Autodesk Fusion 360 part; units mm, degrees
(part 2 of 5)
sketch "Sketch1 (8)" plane through (0, 0, 0) normal (0, 0, 1) x (1, 0, 0) in component "main-switchbody (2)"
  line L0 (0, 0) -> (0, 20) construction
  line L1 (0, 20) -> (20, 20) construction
  line L2 (20, 20) -> (20, 0) construction
  line L3 (20, 0) -> (0, 0) construction
  line L4 (0, 0) -> (20, 20) construction
  line L5 (20, 0) -> (0, 20) construction
  line L6 (10, 0) -> (18.9, 0) construction
  line L7 (10, 10) -> (18.9, 10) construction
  line L8 (18.9, 10) -> (18.9, 18.9) construction
  line L9 (18.9, 18.9) -> (1.1, 18.9) construction
  line L10 (1.1, 18.9) -> (1.1, 1.1) construction
  line L11 (1.1, 1.1) -> (18.9, 1.1) construction
  line L12 (18.9, 1.1) -> (18.9, 18.9) construction
  line L13 (10, 10) -> (3.05, 10) construction
  line L14 (3.05, 10) -> (3.05, 16.95) construction
  line L15 (3.05, 16.95) -> (16.95, 16.95) construction
  line L16 (16.95, 16.95) -> (16.95, 3.05) construction
  line L17 (16.95, 3.05) -> (3.05, 3.05) construction
  line L18 (3.05, 3.05) -> (3.05, 16.95) construction
  line L19 (3.05, 3.05) -> (0, 3.05) construction
  line L20 (3.05, 3.05) -> (3.05, 0) construction
  line L21 (16.95, 3.05) -> (20, 3.05) construction
  line L22 (16.95, 16.95) -> (20, 16.95) construction
  line L23 (16.95, 16.95) -> (16.95, 20) construction
  line L24 (3.05, 16.95) -> (3.05, 20) construction
  line L25 (3.05, 16.95) -> (0, 16.95) construction
  line L26 (3.05, 18.9) -> (6.05, 18.9) construction
  line L27 (6.05, 18.9) -> (6.05, 20) construction
  line L28 (16.95, 18.9) -> (13.95, 18.9) construction
  line L29 (13.95, 18.9) -> (13.95, 20) construction
  line L30 (16.95, 3.05) -> (16.95, 0) construction
  line L31 (16.95, 1.1) -> (13.95, 1.1) construction
  line L32 (13.95, 1.1) -> (13.95, 0) construction
  line L33 (3.05, 1.1) -> (6.05, 1.1) construction
  line L34 (6.05, 1.1) -> (6.05, 0) construction
  line L35 (0, 20) -> (20, 20) construction
  line L36 (20, 20) -> (20, 0) construction
  line L37 (20, 0) -> (0, 0) construction
  line L38 (0, 0) -> (0, 20) construction
  line L39 (0, 20) -> (20, 20)
  line L40 (20, 20) -> (20, 0)
  line L41 (20, 0) -> (0, 0)
  line L42 (0, 0) -> (0, 20)
  line L43 (16.95, 3.05) -> (3.05, 3.05)
  line L44 (3.05, 3.05) -> (3.05, 16.95)
  line L45 (3.05, 16.95) -> (16.95, 16.95)
  line L46 (16.95, 16.95) -> (16.95, 3.05)
  line L47 (3.05, 1.1) -> (6.05, 1.1)
  line L48 (6.05, 1.1) -> (6.05, 0)
  line L49 (6.05, 0) -> (3.05, 0)
  line L50 (3.05, 0) -> (3.05, 1.1)
  line L51 (13.95, 1.1) -> (16.95, 1.1)
  line L52 (16.95, 1.1) -> (16.95, 0)
  line L53 (16.95, 0) -> (13.95, 0)
  line L54 (13.95, 0) -> (13.95, 1.1)
  line L55 (13.95, 20) -> (16.95, 20)
  line L56 (16.95, 20) -> (16.95, 18.9)
  line L57 (16.95, 18.9) -> (13.95, 18.9)
  line L58 (13.95, 18.9) -> (13.95, 20)
  line L59 (3.05, 20) -> (6.05, 20)
  line L60 (6.05, 20) -> (6.05, 18.9)
  line L61 (6.05, 18.9) -> (3.05, 18.9)
  line L62 (3.05, 18.9) -> (3.05, 20)
  line L63 (1.1, 10) -> (1.1, 12)
  line L64 (1.1, 10) -> (1.1, 8)
  line L65 (1.1, 8) -> (-1.9, 8)
  line L66 (-1.9, 8) -> (1.1, 8)
  line L67 (1.1, 8) -> (1.1, 12)
  line L68 (1.1, 12) -> (-1.9, 12)
  line L69 (-1.9, 12) -> (-1.9, 8)
  line L70 (3.05, 10) -> (3.05, 7.5) construction
  line L71 (3.05, 7.5) -> (2.55, 7.5) construction
  line L72 (2.55, 7.5) -> (2.55, 12.5) construction
  line L73 (2.55, 12.5) -> (3.05, 12.5085) construction
  line L74 (3.05, 12.5085) -> (3.05, 7.5) construction
  line L75 (2.55, 12.5) -> (16.95, 12.5) construction
  line L76 (16.95, 12.5) -> (17.45, 12.5) construction
  line L77 (17.45, 12.5) -> (17.45, 7.5) construction
  line L78 (17.45, 7.5) -> (16.95, 7.5) construction
  line L79 (16.95, 7.5) -> (16.95, 12.5) construction
  line L80 (17.45, 7.5) -> (16.95, 7.5)
  line L81 (16.95, 7.5) -> (16.95, 12.5)
  line L82 (16.95, 12.5) -> (17.45, 12.5)
  line L83 (17.45, 12.5) -> (17.45, 7.5)
  line L84 (3.05, 7.5) -> (2.55, 7.5)
  line L85 (2.55, 7.5) -> (2.55, 12.5)
  line L86 (2.55, 12.5) -> (3.05, 12.5)
  line L87 (3.05, 12.5) -> (3.05, 7.5)
  dimension "d1_2" = 20
  dimension "d2_2" = 20
  dimension "d3_2" = 8.9
  dimension "d4_2" = 8.9
  dimension "d5_2" = 8.9
  dimension "d6_2" = 17.8
  dimension "d7_2" = 17.8
  dimension "d8_2" = 6.95
  dimension "d9_2" = 6.95
  dimension "d10_2" = 13.9
  dimension "d11_2" = 13.9
  dimension "d12_2" = 13.9
  dimension "d13_2" = 3
  dimension "d14_2" = 3
  dimension "d15_2" = 3
  dimension "d16_2" = 3
  dimension "d21_4" = 3
  dimension "d58_4" = 2.5
  dimension "d59_4" = 0.5
  dimension "d60_4" = 5
  dimension "d61_4" = 0.5
  dimension "d62_4" = 5
  constraint coincident L0.start L3.end
  constraint vertical L0
  constraint perpendicular L0 L1
  constraint perpendicular L1 L2
  constraint perpendicular L0 L3
  constraint midpoint L3 L6.start
  constraint parallel L3 L6
  constraint midpoint L4 L7.start
  constraint parallel L6 L7
  constraint perpendicular L7 L8
  constraint perpendicular L8 L9
  constraint perpendicular L9 L10
  constraint coincident L5 L11.end
  constraint perpendicular L10 L11
  constraint perpendicular L12 L13
  constraint perpendicular L13 L14
  constraint perpendicular L14 L15
  constraint perpendicular L7 L16
  constraint perpendicular L16 L17
  constraint coincident L0 L19.end
  constraint perpendicular L0 L19
  constraint coincident L3 L20.end
  constraint perpendicular L3 L20
  constraint coincident L2 L21.end
  constraint perpendicular L2 L21
  constraint coincident L2 L22.end
  constraint perpendicular L2 L22
  constraint coincident L1 L23.end
  constraint perpendicular L1 L23
  constraint coincident L1 L24.end
  constraint perpendicular L1 L24
  constraint coincident L0 L25.end
  constraint perpendicular L0 L25
  constraint coincident L24 L26.start
  constraint coincident L9 L26.start
  constraint coincident L9 L26.end
  constraint coincident L1 L27.end
  constraint perpendicular L1 L27
  constraint coincident L9 L28.start
  constraint coincident L23 L28.start
  constraint perpendicular L23 L28
  constraint coincident L1 L29.end
  constraint perpendicular L1 L29
  constraint coincident L6 L30.end
  constraint coincident L30 L31.start
  constraint coincident L11 L31.start
  constraint perpendicular L30 L31
  constraint coincident L6 L32.end
  constraint coincident L11 L33.start
  constraint coincident L20 L33.start
  constraint perpendicular L20 L33
  constraint coincident L3 L34.end
  constraint perpendicular L3 L34
  constraint horizontal L35
  constraint vertical L36
  constraint horizontal L37
  constraint vertical L38
  constraint horizontal L39
  constraint vertical L40
  constraint horizontal L41
  constraint vertical L42
  constraint horizontal L43
  constraint vertical L44
  constraint horizontal L45
  constraint vertical L46
  constraint horizontal L47
  constraint vertical L48
  constraint horizontal L49
  constraint vertical L50
  constraint horizontal L51
  constraint vertical L52
  constraint horizontal L53
  constraint vertical L54
  constraint horizontal L55
  constraint vertical L56
  constraint horizontal L57
  constraint vertical L58
  constraint horizontal L59
  constraint vertical L60
  constraint horizontal L61
  constraint vertical L62
  constraint midpoint L10 L63.start
  constraint coincident L10 L63.end
  constraint parallel L10 L63
  constraint coincident L10 L64.end
  constraint perpendicular L0 L65
  constraint horizontal L66
  constraint vertical L67
  constraint horizontal L68
  constraint vertical L69
  constraint perpendicular L13 L70
  constraint perpendicular L70 L71
  constraint perpendicular L71 L72
  constraint coincident L14 L73.end
  constraint perpendicular L71 L74
  constraint coincident L16 L75.end
  constraint perpendicular L16 L75
  constraint perpendicular L16 L76
  constraint perpendicular L76 L77
  constraint coincident L16 L78.end
  constraint perpendicular L16 L78
  constraint horizontal L80
  constraint vertical L81
  constraint horizontal L82
  constraint vertical L83
  constraint horizontal L84
  constraint vertical L85
  constraint horizontal L86
  constraint vertical L87
  measures "d1_2" distance of L0.start L0.end
  measures "d2_2" distance of L0.end L1.end
  measures "d3_2" distance of L6.start L6.end
  measures "d4_2" distance of L7.start L7.end
  measures "d5_2" distance of L7.end L8.end
  measures "d6_2" distance of L8.end L9.end
  measures "d7_2" distance of L9.end L10.end
  measures "d8_2" distance of L7.start L13.end
  measures "d9_2" distance of L13.end L14.end
  measures "d10_2" distance of L14.end L15.end
  measures "d11_2" distance of L15.end L16.end
  measures "d12_2" distance of L16.end L17.end
  measures "d13_2" distance of L26.start L26.end
  measures "d14_2" distance of L28.start L28.end
  measures "d15_2" distance of L31.start L31.end
  measures "d16_2" distance of L33.start L33.end
  measures "d21_4" distance of L64.end L65.end
  measures "d58_4" distance of L13.end L70.end
  measures "d59_4" distance of L70.end L71.end
  measures "d60_4" distance of L71.end L72.end
  measures "d61_4" distance of L75.end L76.end
  measures "d62_4" distance of L76.end L77.end
extrude "Extrude3'''" add sketch "Sketch1 (8)" along normal blind 7.5 separate body contours L42 L63 L64 L65 L66 L67 L68 | L42 L65 L66 L68 L69 makes body 11 in component "main-switchbody (2)"
extrude "Extrude2'''" add sketch "Sketch1 (8)" along normal blind 4 separate body contours L39 L40 L41 L42 L47 L48 L50 L51 L52 L54 L56 L57 L58 L60 L61 L62 L63 L64 L65 L66 L67 L68 | L42 L63 L64 L65 L66 L67 L68 | L46 L80 L81 L82 L83 | L44 L84 L85 L86 L87 makes body 12 in component "main-switchbody (2)"
extrude "Extrude1'''''" add sketch "Sketch1 (8)" along normal blind 6 separate body contours L39 L59 L60 L61 L62 | L39 L55 L56 L57 L58 | L41 L47 L48 L49 L50 | L41 L51 L52 L53 L54 makes body 13 at (4.05, 1.1, 2) makes body 14 at (5.05, 20, 4) makes body 15 at (14.95, 1.1, 2) makes body 16 at (14.95, 20, 2) in component "main-switchbody (2)"
extrude "Extrude4'" cut sketch "Sketch1 (8)" along normal blind 2 contours L42 L65 L66 L68 L69 bodies 11 in component "main-switchbody (2)"
sketch "Sketch2 (6)" plane through (1.1, 0, 0) normal (1, 0, 0) x (0, 1, 0) in component "main-switchbody (2)"
  line L0 (8, 0) -> (12, 0)
  line L1 (12, 0) -> (12, 7.5)
  line L2 (12, 7.5) -> (8, 7.5)
  line L3 (8, 7.5) -> (8, 0)
  line L4 (8, 7.5) -> (8, 4) construction
  line L5 (8, 4) -> (12, 4) construction
  line L6 (12, 4) -> (12, 7.5) construction
  line L7 (12, 7.5) -> (8, 7.5) construction
  line L8 (8, 7.5) -> (8, 5.75) construction
  line L9 (8, 5.75) -> (12, 5.75) construction
  line L10 (8, 7.5) -> (12, 7.5)
  line L11 (12, 7.5) -> (12, 5.75)
  line L12 (12, 5.75) -> (8, 5.75)
  line L13 (8, 5.75) -> (8, 7.5)
  dimension "d26_4" = 1.75
  constraint coincident L2.end L3.start
  constraint coincident L3 L4.end
  constraint perpendicular L2 L4
  constraint coincident L1 L5.end
  constraint perpendicular L1 L5
  constraint coincident L1.end L2.start
  constraint perpendicular L2 L6
  constraint perpendicular L5 L8
  constraint midpoint L6 L9.end
  constraint horizontal L10
  constraint vertical L11
  constraint horizontal L12
  constraint vertical L13
  measures "d26_4" distance of L2.end L8.end
extrude "Extrude5'" add sketch "Sketch2 (6)" along normal blind 1 contours L1 L2 L3 L10 L11 L12 L13 bodies 11 in component "main-switchbody (2)"
extrude "Extrude6'" cut 1 faces at (-1.9, 10.6667, 3.8333) along direction (1, 0, 0) blind 1 on bodies 11 bodies 11 in component "main-switchbody (2)"
sketch "Sketch3 (2)" plane through (0, 18.9, 0) normal (0, -1, 0) x (1, 0, 0) in component "main-switchbody (2)"
  line L0 (3.05, 0) -> (6.05, 0)
  line L1 (6.05, 0) -> (6.05, 6)
  line L2 (6.05, 6) -> (3.05, 6)
  line L3 (3.05, 6) -> (3.05, 0)
  line L4 (3.05, 6) -> (3.05, 4) construction
  line L5 (6.05, 4) -> (6.05, 6) construction
  line L6 (3.05, 6) -> (3.05, 4.5) construction
  line L7 (6.05, 6) -> (6.05, 4.5) construction
  arc A0 (6.05, 4.5) -> (3.05, 4.5) centre (4.55, 4.5) ccw construction
  arc A1 (6.05, 4.5) -> (3.05, 4.5) centre (4.55, 4.5) ccw
  dimension "d31_4" = 1.5
  dimension "d32_4" = 1.5
  constraint coincident L2.end L3.start
  constraint coincident L3 L4.end
  constraint perpendicular L2 L4
  constraint coincident L1 L5.start
  constraint coincident L1.end L2.start
  constraint perpendicular L2 L5
  constraint perpendicular L2 L6
  constraint perpendicular L2 L7
  constraint tangent L2 A0
  constraint tangent L2 A1
  measures "d31_4" distance of L2.end L6.end
  measures "d32_4" distance of L1.end L7.end
extrude "Extrude7'" cut sketch "Sketch3 (2)" against normal blind 1.1 contours L2 L3 A1 | L1 L2 A1 bodies 14 in component "main-switchbody (2)"
sketch "Sketch4 (2)" plane through (0, 0, 0) normal (0, -1, 0) x (1, 0, 0) in component "main-switchbody (2)"
  line L0 (3.05, 0) -> (6.05, 0)
  line L1 (6.05, 0) -> (6.05, 6)
  line L2 (6.05, 6) -> (3.05, 6)
  line L3 (3.05, 6) -> (3.05, 0)
  line L4 (3.05, 6) -> (3.05, 4.5) construction
  line L5 (6.05, 6) -> (6.05, 4.5) construction
  arc A0 (6.05, 4.5) -> (3.05, 4.5) centre (4.55, 4.5) ccw
  constraint coincident L2.end L3.start
  constraint coincident L3 L4.end
  constraint perpendicular L2 L4
  constraint coincident L1.end L2.start
  constraint coincident L1 L5.end
  constraint perpendicular L2 L5
  constraint tangent L2 A0
extrude "Extrude8'" cut sketch "Sketch4 (2)" against normal blind 1.1 contours L2 L3 A0 | L1 L2 A0 bodies 13 in component "main-switchbody (2)"
sketch "Sketch5 (2)" plane through (0, 0, 0) normal (0, -1, 0) x (1, 0, 0) in component "main-switchbody (2)"
  line L0 (13.95, 0) -> (16.95, 0)
  line L1 (16.95, 0) -> (16.95, 6)
  line L2 (16.95, 6) -> (13.95, 6)
  line L3 (13.95, 6) -> (13.95, 0)
  line L4 (13.95, 6) -> (13.95, 4.5) construction
  line L5 (16.95, 6) -> (16.95, 4.5) construction
  arc A0 (16.95, 4.5) -> (13.95, 4.5) centre (15.45, 4.5) ccw
  constraint coincident L2.end L3.start
  constraint coincident L3 L4.end
  constraint perpendicular L2 L4
  constraint coincident L1.end L2.start
  constraint coincident L1 L5.end
  constraint perpendicular L2 L5
  constraint tangent L2 A0
extrude "Extrude9'" cut sketch "Sketch5 (2)" against normal blind 1.1 contours L2 L3 A0 | L1 L2 A0 bodies 15 in component "main-switchbody (2)"
sketch "Sketch6 (2)" plane through (0, 18.9, 0) normal (0, -1, 0) x (1, 0, 0) in component "main-switchbody (2)"
  line L0 (13.95, 0) -> (16.95, 0)
  line L1 (16.95, 0) -> (16.95, 6)
  line L2 (16.95, 6) -> (13.95, 6)
  line L3 (13.95, 6) -> (13.95, 0)
  line L4 (13.95, 6) -> (13.95, 4.5) construction
  line L5 (16.95, 6) -> (16.95, 4.5) construction
  arc A0 (16.95, 4.5) -> (13.95, 4.5) centre (15.45, 4.5) ccw
  constraint coincident L2.end L3.start
  constraint coincident L3 L4.end
  constraint perpendicular L2 L4
  constraint coincident L1.end L2.start
  constraint coincident L1 L5.end
  constraint perpendicular L2 L5
  constraint tangent L2 A0
extrude "Extrude10'" cut sketch "Sketch6 (2)" against normal blind 1.1 contours L2 L3 A0 | L1 L2 A0 bodies 16 in component "main-switchbody (2)"
sketch "Sketch7 (2)" plane through (0, 0, 4) normal (0, 0, 1) x (-1, 0, 0) in component "main-switchbody (2)"
  line L0 (-3.05, -16.95) -> (-16.95, -16.95)
  line L1 (-16.95, -16.95) -> (-16.95, -3.05)
  line L2 (-16.95, -3.05) -> (-3.05, -3.05)
  line L3 (-3.05, -3.05) -> (-3.05, -16.95)
  line L4 (-6.05, -20) -> (-6.05, -18.9)
  line L5 (-6.05, -18.9) -> (-3.05, -18.9)
  line L6 (-3.05, -18.9) -> (-3.05, -20)
  line L7 (-3.05, -20) -> (0, -20)
  line L8 (0, -20) -> (0, 0)
  line L9 (0, 0) -> (-3.05, 0)
  line L10 (-3.05, 0) -> (-3.05, -1.1)
  line L11 (-3.05, -1.1) -> (-6.05, -1.1)
  line L12 (-6.05, -1.1) -> (-6.05, 0)
  line L13 (-6.05, 0) -> (-13.95, 0)
  line L14 (-13.95, 0) -> (-13.95, -1.1)
  line L15 (-13.95, -1.1) -> (-16.95, -1.1)
  line L16 (-16.95, -1.1) -> (-16.95, 0)
  line L17 (-16.95, 0) -> (-20, 0)
  line L18 (-20, 0) -> (-20, -20)
  line L19 (-20, -20) -> (-16.95, -20)
  line L20 (-16.95, -20) -> (-16.95, -18.9)
  line L21 (-16.95, -18.9) -> (-13.95, -18.9)
  line L22 (-13.95, -18.9) -> (-13.95, -20)
  line L23 (-13.95, -20) -> (-6.05, -20)
  line L24 (-20, -10) -> (-20, -11.5) construction
  line L25 (-20, -10) -> (-20, -8.5) construction
  line L26 (-20, -8.5) -> (-19, -8.5) construction
  line L27 (-19, -8.5) -> (-19, -11.5) construction
  line L28 (-19, -11.5) -> (-20, -11.5) construction
  line L29 (-20, -11.5) -> (-21, -11.5) construction
  line L30 (-21, -11.5) -> (-21, -8.5) construction
  line L31 (-21, -8.5) -> (-20, -8.5) construction
  line L32 (-19, -11.5) -> (-21, -11.5)
  line L33 (-21, -11.5) -> (-21, -8.5)
  line L34 (-21, -8.5) -> (-19, -8.5)
  line L35 (-19, -8.5) -> (-19, -11.5)
  dimension "d41_4" = 1.5
  dimension "d42_4" = 1
  constraint midpoint L18 L24.start
  constraint parallel L18 L24
  constraint coincident L18 L25.end
  constraint parallel L18 L25
  constraint perpendicular L25 L26
  constraint perpendicular L26 L27
  constraint perpendicular L24 L29
  constraint perpendicular L29 L30
  constraint horizontal L32
  constraint vertical L33
  constraint horizontal L34
  constraint vertical L35
  measures "d41_4" distance of L24.start L24.end
  measures "d42_4" distance of L24.end L29.end
extrude "Extrude11'" add sketch "Sketch7 (2)" along normal blind 3 contours L18 L32 L33 L34 | L18 L32 L34 L35 bodies 12 in component "main-switchbody (2)"
extrude "Extrude12'" add 1 faces at (20, 8.5, 6) along direction (0, -1, 0) blind 0.5 on bodies 12 bodies 12 in component "main-switchbody (2)"
extrude "Extrude13'" add 1 faces at (20, 11.5, 6) along direction (0, 1, 0) blind 0.5 on bodies 12 bodies 12 in component "main-switchbody (2)"
extrude "Extrude14'" add 1 faces at (20.3333, 10.6667, 7) along direction (0, 0, 1) blind 0.75 on bodies 12 bodies 12 in component "main-switchbody (2)"
sketch "Sketch8 (2)" plane through (0, 0, 4) normal (0, 0, -1) x (1, 0, 0) in component "main-switchbody (2)"
  line L0 (20, -8) -> (20, -12)
  line L1 (20, -12) -> (21, -12)
  line L2 (21, -12) -> (21, -8)
  line L3 (21, -8) -> (20, -8)
  line L4 (20, -12) -> (20, -8)
  constraint coincident L0.end L1.start
  constraint coincident L0.start L3.end
extrude "Extrude15'" add sketch "Sketch8 (2)" along normal blind 2 bodies 12 in component "main-switchbody (2)"
sketch "Sketch9 (3)" plane through (19, 0, 0) normal (-1, 0, 0) x (0, -1, 0) in component "main-switchbody (2)"
  line L0 (-12, 4) -> (-8, 4)
  line L1 (-8, 4) -> (-8, 7.75)
  line L2 (-8, 7.75) -> (-12, 7.75)
  line L3 (-12, 7.75) -> (-12, 4)
  line L4 (-12, 7.75) -> (-12, 5.75) construction
  line L5 (-12, 5.75) -> (-8, 5.75) construction
  line L6 (-12, 7.75) -> (-8, 7.75)
  line L7 (-8, 7.75) -> (-8, 5.75)
  line L8 (-8, 5.75) -> (-12, 5.75)
  line L9 (-12, 5.75) -> (-12, 7.75)
  dimension "d53_4" = 2
  constraint coincident L2.end L3.start
  constraint perpendicular L2 L4
  constraint coincident L1 L5.end
  constraint perpendicular L1 L5
  constraint horizontal L6
  constraint vertical L7
  constraint horizontal L8
  constraint vertical L9
  measures "d53_4" distance of L2.end L4.end
extrude "Extrude16'" add sketch "Sketch9 (3)" along normal blind 0.5 contours L1 L2 L3 L6 L7 L8 L9 bodies 12 in component "main-switchbody (2)"
extrude "Extrude17'" cut 1 faces at (2.1, 9.3333, 6.9167) along direction (-1, 0, 0) blind 0.3 on bodies 11 bodies 11 in component "main-switchbody (2)"
extrude "Extrude18'" cut sketch "Sketch1 (8)" along normal blind 2.7 contours L44 L84 L85 L86 L87 bodies 12 in component "main-switchbody (2)"
extrude "Extrude19'" cut sketch "Sketch1 (8)" along normal blind 2.7 contours L46 L80 L81 L82 L83 bodies 12 in component "main-switchbody (2)"
extrude "Extrude20'" add sketch "Sketch1 (8)" against normal blind 0.2 contours L39 L40 L41 L42 L47 L48 L50 L51 L52 L54 L56 L57 L58 L60 L61 L62 L63 L64 L65 L66 L67 L68 | L39 L59 L60 L61 L62 | L42 L63 L64 L65 L66 L67 L68 | L39 L55 L56 L57 L58 | L41 L47 L48 L49 L50 | L41 L51 L52 L53 L54 bodies 11 12 13 14 15 16 in component "main-switchbody (2)"
fillet "Fillet1'" radius 1 2 edges at (21, 10, 7.75) (-0.9, 10, 7.5) on bodies 11 12 in component "main-switchbody (2)"
extrude "Extrude21'" add 1 faces at (2.8833, 9.1667, 2.7) along direction (0, 0, -1) blind 2.9 on bodies 11 bodies 11 in component "main-switchbody (2)"
extrude "Extrude22'" add 1 faces at (17.1167, 10.8333, 2.7) along direction (0, 0, -1) blind 2.9 on bodies 11 bodies 11 in component "main-switchbody (2)"
sketch "Sketch10 (2)" plane through (0, 0, 4) normal (0, 0, 1) x (-1, 0, 0) in component "main-switchbody (2)"
  line L0 (-3.05, -16.95) -> (-16.95, -16.95)
  line L1 (-16.95, -16.95) -> (-16.95, -3.05)
  line L2 (-16.95, -3.05) -> (-3.05, -3.05)
  line L3 (-3.05, -3.05) -> (-3.05, -16.95)
  line L4 (0, -12) -> (-1.1, -12)
  line L5 (-1.1, -12) -> (-1.1, -8)
  line L6 (-1.1, -8) -> (0, -8)
  line L7 (0, -8) -> (0, 0)
  line L8 (0, 0) -> (-3.05, 0)
  line L9 (-3.05, 0) -> (-3.05, -1.1)
  line L10 (-3.05, -1.1) -> (-6.05, -1.1)
  line L11 (-6.05, -1.1) -> (-6.05, 0)
  line L12 (-6.05, 0) -> (-13.95, 0)
  line L13 (-13.95, 0) -> (-13.95, -1.1)
  line L14 (-13.95, -1.1) -> (-16.95, -1.1)
  line L15 (-16.95, -1.1) -> (-16.95, 0)
  line L16 (-16.95, 0) -> (-20, 0)
  line L17 (-20, 0) -> (-20, -8)
  line L18 (-20, -8) -> (-19, -8)
  line L19 (-19, -8) -> (-19, -12)
  line L20 (-19, -12) -> (-20, -12)
  line L21 (-20, -12) -> (-20, -20)
  line L22 (-20, -20) -> (-16.95, -20)
  line L23 (-16.95, -20) -> (-16.95, -18.9)
  line L24 (-16.95, -18.9) -> (-13.95, -18.9)
  line L25 (-13.95, -18.9) -> (-13.95, -20)
  line L26 (-13.95, -20) -> (-6.05, -20)
  line L27 (-6.05, -20) -> (-6.05, -18.9)
  line L28 (-6.05, -18.9) -> (-3.05, -18.9)
  line L29 (-3.05, -18.9) -> (-3.05, -20)
  line L30 (-3.05, -20) -> (0, -20)
  line L31 (0, -20) -> (0, -12)
  line L32 (-3.05, -10) -> (-3.05, -12.5) construction
  line L33 (-3.05, -12.5) -> (-3.05, -7.5) construction
  line L34 (-3.05, -7.5) -> (-2.55, -7.5) construction
  line L35 (-2.55, -7.5) -> (-3.05, -7.5) construction
  line L36 (-3.05, -7.5) -> (-3.05, -12.5) construction
  line L37 (-3.05, -12.5) -> (-2.55, -12.5) construction
  line L38 (-2.55, -12.5) -> (-2.55, -7.5) construction
  line L39 (-3.05, -12.5) -> (-16.95, -12.5) construction
  line L40 (-16.95, -12.5) -> (-16.95, -7.5) construction
  line L41 (-16.95, -7.5) -> (-17.45, -7.5) construction
  line L42 (-17.45, -7.5) -> (-16.95, -7.5) construction
  line L43 (-16.95, -7.5) -> (-16.95, -12.5) construction
  line L44 (-16.95, -12.5) -> (-17.45, -12.5) construction
  line L45 (-17.45, -12.5) -> (-17.45, -7.5) construction
  line L46 (-16.95, -12.5) -> (-17.45, -12.5)
  line L47 (-17.45, -12.5) -> (-17.45, -7.5)
  line L48 (-17.45, -7.5) -> (-16.95, -7.5)
  line L49 (-16.95, -7.5) -> (-16.95, -12.5)
  line L50 (-2.55, -12.5) -> (-3.05, -12.5)
  line L51 (-3.05, -12.5) -> (-3.05, -7.5)
  line L52 (-3.05, -7.5) -> (-2.55, -7.5)
  line L53 (-2.55, -7.5) -> (-2.55, -12.5)
  dimension "d75_2" = 5
  dimension "d76_2" = 0.5
  dimension "d77_2" = 0.5
  constraint midpoint L3 L32.start
  constraint coincident L3 L32.end
  constraint perpendicular L0 L32
  constraint parallel L3 L33
  constraint perpendicular L33 L34
  constraint horizontal L35
  constraint vertical L36
  constraint horizontal L37
  constraint vertical L38
  constraint coincident L1 L39.end
  constraint perpendicular L1 L39
  constraint coincident L1 L40.end
  constraint perpendicular L39 L40
  constraint perpendicular L40 L41
  constraint horizontal L42
  constraint vertical L43
  constraint horizontal L44
  constraint vertical L45
  constraint horizontal L46
  constraint vertical L47
  constraint horizontal L48
  constraint vertical L49
  constraint horizontal L50
  constraint vertical L51
  constraint horizontal L52
  constraint vertical L53
  measures "d75_2" distance of L32.end L33.end
  measures "d76_2" distance of L33.end L34.end
  measures "d77_2" distance of L40.end L41.end
extrude "Extrude23'" cut sketch "Sketch10 (2)" against normal blind 2.9 contours L3 L50 L51 L52 L53 | L1 L46 L47 L48 L49 bodies 11 in component "main-switchbody (2)"
extrude "Extrude24'" cut 2 faces at (4.8122, 18.9, 5.1079) (15.1626, 18.9, 5.4316) along direction (0, 1, 0) blind 0.25 on bodies 11 bodies 11 in component "main-switchbody (2)"
extrude "Extrude25'" cut 2 faces at (4.2822, 1.1, 5.1824) (15.2673, 1.1, 4.9654) along direction (0, -1, 0) blind 0.25 on bodies 11 bodies 11 in component "main-switchbody (2)"
extrude "Extrude26'" add 1 faces at (1.0167, 12.3167, -0.2) along direction (0, 0, -1) blind 1 on bodies 11 bodies 11 in component "main-switchbody (2)"
extrude "Extrude27'" cut 1 faces at (1.0167, 12.3167, -1.2) along direction (0, 0, 1) blind 0.2 on bodies 11 bodies 11 in component "main-switchbody (2)"
extrude "Extrude28'" cut 2 faces at (17.1167, 10.8333, 1.1) (2.8833, 9.1667, 1.1) along direction (0, 0, -1) blind 0.8 on bodies 11 bodies 11 in component "main-switchbody (2)"
extrude "Extrude29'" cut 1 faces at (18.8333, 9.3333, 5.75) along direction (0, 0, 1) blind 0.2 on bodies 11 bodies 11 in component "main-switchbody (2)"
extrude "Extrude30'" cut 1 faces at (1.3333, 10.6667, 5.75) along direction (0, 0, 1) blind 0.2 on bodies 11 bodies 11 in component "main-switchbody (2)"
sketch "Sketch1 (9)" plane through (0, 0, 0.0152) normal (0, 0, -1) x (1, 0, 0) in component "mxledbit-switchbody v10 (2)"
  line L0 (4.5419, -16.2374) -> (4.5419, -2.3374)
  line L1 (4.5419, -2.3374) -> (18.4419, -2.3374)
  line L2 (18.4419, -2.3374) -> (18.4419, -16.2374)
  line L3 (18.4419, -16.2374) -> (4.5419, -16.2374)
  line L4 (1.4919, -19.2874) -> (21.4919, -19.2874)
  line L5 (21.4919, -19.2874) -> (21.4919, 0.7126)
  line L6 (21.4919, 0.7126) -> (1.4919, 0.7126)
  line L7 (1.4919, 0.7126) -> (1.4919, -19.2874)
ref_plane "WorkPlane1" through (5, 31.8794, 9.316) normal (0, -0.939693, 0.34202) x (1, 0, 0) in component "wheel (1)"
sketch "Sketch2 (7)" plane through (5, 31.8794, 9.316) normal (0, -0.939693, 0.34202) x (1, 0, 0) in component "wheel (1)"
  circle A0 centre (0, 0) radius 80
  dimension "d64_1" = 160
  constraint coincident A0.centre origin
  measures "d64_1" diameter of A0
component_pattern "component pattern'" in component "Index2"
sketch "Sketch2 (8)" plane through (0, 23.2767, -8.472) normal (0, -0.939693, 0.34202) x (1, 0, 0) in component "IND-Sketch (1)"
  circle A0 centre (5, 19.6575) radius 80
  line L0 (5, 19.6575) -> (5, -60.3425) construction
  line L1 (5, -60.3425) -> (-10, -60.3425) construction
  line L2 (-10, -60.3425) -> (20, -60.3425)
  line L3 (20, -60.3425) -> (20, 19.6575)
  line L4 (20, 19.6575) -> (-10, 19.6575)
  line L5 (-10, 19.6575) -> (-10, -60.3425)
  dimension "d69_1" = 80
  dimension "d70_1" = 15
  dimension "d71_1" = 30
  dimension "d72_1" = 80
  constraint coincident A0.centre L0.start
  constraint vertical L0
  constraint perpendicular L0 L1
  constraint horizontal L2
  constraint vertical L3
  constraint horizontal L4
  constraint vertical L5
  measures "d69_1" distance of A0.centre L0.end
  measures "d70_1" distance of L0.end L1.end
  measures "d71_1" distance of L1.end L2.end
  measures "d72_1" distance of L1.end L4.end
sketch "Sketch9 (4)" plane through (5, 41.9534, 55.6343) normal (0, 0.573576, 0.819152) x (-1, 0, 0) in component "IND-Sketch (1)"
  line L0 (-45, -9.823) -> (5, -9.823) construction
  line L1 (-20, -9.823) -> (5, -9.823) construction
  line L2 (-20, -9.823) -> (-45, -9.823) construction
  circle A0 centre (-20, -9.823) radius 75 construction
  point P0 (-20, -9.823)
  point P1 (-45, -9.823)
  point P2 (5, -9.823)
  point P3 (5, -9.823)
  point P4 (-45, -9.823)
  dimension "d38_1" = 30
  dimension "d39_1" = 15
  dimension "d40_1" = 15
  dimension "d41_1" = 160
  constraint coincident P4 P1
  constraint horizontal L0
  constraint coincident P0 L1.start
  constraint parallel L0 L1
  constraint parallel L0 L2
sketch "Sketch1 (10)" plane through (0, 54.7581, -45.9475) normal (0, -0.766044, 0.642788) x (1, 0, 0) in component "IND-Sketch (1)"
  line L0 (-1.3269, 70.632) -> (-1.3269, 84.532)
  line L1 (-1.3269, 84.532) -> (12.5731, 84.532)
  line L2 (12.5731, 84.532) -> (12.5731, 70.632)
  line L3 (12.5731, 70.632) -> (-1.3269, 70.632)
  line L4 (-4.3769, 67.582) -> (15.6231, 67.582)
  line L5 (15.6231, 67.582) -> (15.6231, 87.582)
  line L6 (15.6231, 87.582) -> (-4.3769, 87.582)
  line L7 (-4.3769, 87.582) -> (-4.3769, 67.582)
  line L8 (-4.3769, 77.582) -> (15.6231, 77.582) construction
  line L9 (5.6231, 87.582) -> (5.6231, 67.582) construction
  point P0 (5.6231, 77.582)
  constraint midpoint L7 L8.start
  constraint midpoint L5 L8.end
  constraint midpoint L6 L9.start
  constraint midpoint L4 L9.end
  constraint midpoint L8 P0
ref_plane "WorkPlane2" through (0, 34, 0) normal (0, 1, 0) x (0, 0, 1) in component "IND-Sketch (2)"
sketch "IND-originXY (3)" plane through (0, 0, 0) normal (0, 0, 1) x (1, 0, 0) in component "IND-Sketch (2)"
  line L0 (0, 0) -> (0, 16) construction
  line L1 (0, 16) -> (16, 16) construction
  line L2 (16, 16) -> (16, -18) construction
  line L3 (16, -18) -> (-18, -18) construction
  line L4 (0, 16) -> (17, 16) construction
  point P0 (17, 16)
  dimension "d20_3" = 16
  dimension "d21_3" = 16
  dimension "d29_3" = 34
  dimension "d30_3" = 34
  dimension "d34_3" = 17
  constraint coincident L0.start origin
  constraint vertical L0
  constraint perpendicular L0 L1
  constraint perpendicular L1 L2
  constraint perpendicular L0 L3
  constraint perpendicular L0 L4
  constraint coincident P0 L4.end
  measures "d20_3" distance of L0.start L0.end
  measures "d21_3" distance of L0.end L1.end
  measures "d29_3" distance of L1.end L2.end
  measures "d30_3" distance of L2.end L3.end
  measures "d34_3" distance of L0.end P0
sketch "IND-originXZ (3)" plane through (0, 34, 0) normal (0, 1, 0) x (1, 0, 0) in component "IND-Sketch (2)"
  line L0 (0, 0) -> (16, 0) construction
  line L1 (10, 0) -> (10, -10) construction
  line L2 (10, -10) -> (0, -10) construction
  line L3 (0, -10) -> (0, 0) construction
  line L4 (10, -10) -> (5, -10) construction
  line L5 (0, -10) -> (5, -10) construction
  line L6 (0, -10) -> (5, -10) construction
  point P0 (16, 0)
  point P1 (0, -10)
  point P2 (10, -10)
  point P3 (17, 0)
  point P4 (5, -10)
  dimension "d26_3" = 10
  dimension "d27_3" = 34
  dimension "d28_3" = 34
  dimension "d36_3" = 17
  dimension "d37_3" = 17
  constraint coincident P0 L1.start
  constraint perpendicular L0 L1
  constraint perpendicular L1 L2
  constraint coincident L0.start L3.end
  constraint coincident P1 L2.end
  constraint coincident P2 L1.end
  constraint midpoint L2 P4
  constraint perpendicular L1 L4
  constraint parallel L4 L6
  measures "d26_3" distance of L1.start P2
ref_plane "WorkPlane3" through (5, 34, 10) normal (0, 0.996195, -0.087156) x (-1, 0, 0) in component "IND-Sketch (2)"
sketch "IND-path (3)" plane through (5, 34.1975, 12.2574) normal (0, 0.996195, -0.087156) x (-1, 0, 0) in component "IND-Sketch (2)"
  line L0 (-5, -2.266) -> (5, -2.266) construction
  line L1 (5, -2.266) -> (-5, -2.266) construction
  circle A0 centre (0, 0) radius 85 construction
  line L2 (0, 0) -> (17, 0) construction
  line L3 (0, 0) -> (-17, 0) construction
  line L4 (0, 0) -> (0, -85) construction
  line L5 (0, -85) -> (6.95, -85) construction
  line L6 (0, -85) -> (-6.95, -85) construction
  point P0 (-5, -2.266)
  point P1 (5, -2.266)
  point P2 (0, -85)
  dimension "d32_3" = 170
  dimension "d33_3" = 17
  dimension "d35_3" = 17
  dimension "d42_3" = 85
  dimension "d43_3" = 6.95
  dimension "d44_3" = 6.95
  dimension "d67_3" = 90
  constraint coincident P1 L0.end
  constraint coincident P0 L0.start
  constraint coincident A0.centre L2.start
  constraint parallel L1 L2
  constraint parallel L0 L3
  constraint coincident P2 L4.end
  constraint perpendicular L4 L5
  constraint perpendicular L4 L6
  measures "d32_3" diameter of A0
  measures "d33_3" distance of A0.centre L2.end
  measures "d35_3" distance of A0.centre L3.end
  measures "d42_3" distance of A0.centre P2
  measures "d43_3" distance of P2 L5.end
  measures "d44_3" distance of P2 L6.end
  measures "d67_3" angle of L2 L4
sketch "Sketch1 (11)" plane through (5, 34.1975, 12.2574) normal (0, 0.996195, -0.087156) x (-1, 0, 0) in component "wheel (2)"
  circle A0 centre (0, 0) radius 85
  line L0 (0, -85) -> (6.95, -85)
  line L1 (0, -85) -> (-6.95, -85)
  line L2 (0, -85) -> (0, 85) construction
  line L3 (0, 0) -> (85, 0) construction
  circle A1 centre (0, 0) radius 85
  point P0 (0, -85)
  point P1 (0, -2.266)
  dimension "d45_3" = 170
  dimension "d46_3" = 85
  dimension "d47_3" = 170
  constraint coincident P0 L0.start
  constraint perpendicular L0 L2
  constraint coincident A0.centre L3.start
  constraint perpendicular L2 L3
  measures "d45_3" distance of P0 L2.end
  measures "d46_3" distance of A0.centre L3.end
  measures "d47_3" diameter of A1
extrude "Extrude1''''''" add sketch "Sketch1 (11)" along normal blind 4 separate body makes body 17 in component "wheel (2)"
ref_plane "WorkPlane1" through (5, 50.9494, -74.5329) normal (0, -0.087156, -0.996195) x (1, 0, 0) in component "plug (2)"
sketch "Sketch1 (12)" plane through (5, 73.9095, -76.5416) normal (0, -0.087156, -0.996195) x (1, 0, 0) in component "plug (2)"
  line L0 (-85, 43.3002) -> (85, 43.3002)
  line L1 (-85, 43.3002) -> (85, 43.3002)
  line L2 (-85, 47.3002) -> (85, 47.3002)
  line L3 (-85, 47.3002) -> (85, 47.3002)
  line L4 (0, 47.3002) -> (0, 43.3002) construction
  line L5 (0, 47.3002) -> (-6.95, 47.3002) construction
  line L6 (0, 47.3002) -> (6.95, 47.3002) construction
  line L7 (6.95, 47.3002) -> (6.95, 43.3002) construction
  line L8 (-6.95, 47.3002) -> (-6.95, 43.3002) construction
  line L9 (-6.95, 43.3002) -> (6.95, 43.3002) construction
  line L10 (6.95, 43.3002) -> (-6.95, 43.3002)
  line L11 (-6.95, 43.3002) -> (-6.95, 47.3002)
  line L12 (-6.95, 47.3002) -> (6.95, 47.3002)
  line L13 (6.95, 47.3002) -> (6.95, 43.3002)
  point P0 (0, 47.3002)
  dimension "d51_3" = 6.95
  dimension "d52_3" = 6.95
  constraint coincident P0 L4.start
  constraint midpoint L1 L4.end
  constraint perpendicular L4 L5
  constraint perpendicular L4 L6
  constraint coincident L1 L7.end
  constraint perpendicular L1 L7
  constraint coincident L0 L8.end
  constraint perpendicular L0 L8
  constraint horizontal L10
  constraint vertical L11
  constraint horizontal L12
  constraint vertical L13
  measures "d51_3" distance of P0 L5.end
  measures "d52_3" distance of P0 L6.end
extrude "Extrude1'''''''" add sketch "Sketch1 (12)" along normal blind 4 separate body makes body 18 in component "plug (2)"
sketch "Sketch2 (9)" plane through (0, -6.0842, -69.5431) normal (0, 0.087156, 0.996195) x (1, 0, 0) in component "plug (2)"
  line L0 (-1.95, 32.9991) -> (11.95, 32.9991)
  line L1 (11.95, 32.9991) -> (11.95, 36.9991)
  line L2 (11.95, 36.9991) -> (-1.95, 36.9991)
  line L3 (-1.95, 36.9991) -> (-1.95, 32.9991)
extrude "Extrude2''''" add 1 faces at (2.6833, 30.5416, -75.4243) along direction (0, 0.996195, -0.087156) blind 4.95 on bodies 18 bodies 18 in component "plug (2)"
extrude "Extrude3''''" add 1 faces at (7.3167, 26.5568, -75.0756) along direction (0, -0.996195, 0.087156) blind 4.95 on bodies 18 bodies 18 in component "plug (2)"
sketch "Sketch1 (13)" plane through (0, 0, 0) normal (0, 0, 1) x (1, 0, 0) in component "main-switchbody (3)"
  line L0 (0, 0) -> (0, 20) construction
  line L1 (0, 20) -> (20, 20) construction
  line L2 (20, 20) -> (20, 0) construction
  line L3 (20, 0) -> (0, 0) construction
  line L4 (0, 0) -> (20, 20) construction
  line L5 (20, 0) -> (0, 20) construction
  line L6 (10, 0) -> (18.9, 0) construction
  line L7 (10, 10) -> (18.9, 10) construction
  line L8 (18.9, 10) -> (18.9, 18.9) construction
  line L9 (18.9, 18.9) -> (1.1, 18.9) construction
  line L10 (1.1, 18.9) -> (1.1, 1.1) construction
  line L11 (1.1, 1.1) -> (18.9, 1.1) construction
  line L12 (18.9, 1.1) -> (18.9, 18.9) construction
  line L13 (10, 10) -> (3.05, 10) construction
  line L14 (3.05, 10) -> (3.05, 16.95) construction
  line L15 (3.05, 16.95) -> (16.95, 16.95) construction
  line L16 (16.95, 16.95) -> (16.95, 3.05) construction
  line L17 (16.95, 3.05) -> (3.05, 3.05) construction
  line L18 (3.05, 3.05) -> (3.05, 16.95) construction
  line L19 (3.05, 3.05) -> (0, 3.05) construction
  line L20 (3.05, 3.05) -> (3.05, 0) construction
  line L21 (16.95, 3.05) -> (20, 3.05) construction
  line L22 (16.95, 16.95) -> (20, 16.95) construction
  line L23 (16.95, 16.95) -> (16.95, 20) construction
  line L24 (3.05, 16.95) -> (3.05, 20) construction
  line L25 (3.05, 16.95) -> (0, 16.95) construction
  line L26 (3.05, 18.9) -> (6.05, 18.9) construction
  line L27 (6.05, 18.9) -> (6.05, 20) construction
  line L28 (16.95, 18.9) -> (13.95, 18.9) construction
  line L29 (13.95, 18.9) -> (13.95, 20) construction
  line L30 (16.95, 3.05) -> (16.95, 0) construction
  line L31 (16.95, 1.1) -> (13.95, 1.1) construction
  line L32 (13.95, 1.1) -> (13.95, 0) construction
  line L33 (3.05, 1.1) -> (6.05, 1.1) construction
  line L34 (6.05, 1.1) -> (6.05, 0) construction
  line L35 (0, 20) -> (20, 20) construction
  line L36 (20, 20) -> (20, 0) construction
  line L37 (20, 0) -> (0, 0) construction
  line L38 (0, 0) -> (0, 20) construction
  line L39 (0, 20) -> (20, 20)
  line L40 (20, 20) -> (20, 0)
  line L41 (20, 0) -> (0, 0)
  line L42 (0, 0) -> (0, 20)
  line L43 (16.95, 3.05) -> (3.05, 3.05)
  line L44 (3.05, 3.05) -> (3.05, 16.95)
  line L45 (3.05, 16.95) -> (16.95, 16.95)
  line L46 (16.95, 16.95) -> (16.95, 3.05)
  line L47 (3.05, 1.1) -> (6.05, 1.1)
  line L48 (6.05, 1.1) -> (6.05, 0)
  line L49 (6.05, 0) -> (3.05, 0)
  line L50 (3.05, 0) -> (3.05, 1.1)
  line L51 (13.95, 1.1) -> (16.95, 1.1)
  line L52 (16.95, 1.1) -> (16.95, 0)
  line L53 (16.95, 0) -> (13.95, 0)
  line L54 (13.95, 0) -> (13.95, 1.1)
  line L55 (13.95, 20) -> (16.95, 20)
  line L56 (16.95, 20) -> (16.95, 18.9)
  line L57 (16.95, 18.9) -> (13.95, 18.9)
  line L58 (13.95, 18.9) -> (13.95, 20)
  line L59 (3.05, 20) -> (6.05, 20)
  line L60 (6.05, 20) -> (6.05, 18.9)
  line L61 (6.05, 18.9) -> (3.05, 18.9)
  line L62 (3.05, 18.9) -> (3.05, 20)
  line L63 (1.1, 10) -> (1.1, 12)
  line L64 (1.1, 10) -> (1.1, 8)
  line L65 (1.1, 8) -> (-1.9, 8)
  line L66 (-1.9, 8) -> (1.1, 8)
  line L67 (1.1, 8) -> (1.1, 12)
  line L68 (1.1, 12) -> (-1.9, 12)
  line L69 (-1.9, 12) -> (-1.9, 8)
  line L70 (3.05, 10) -> (3.05, 7.5) construction
  line L71 (3.05, 7.5) -> (2.55, 7.5) construction
  line L72 (2.55, 7.5) -> (2.55, 12.5) construction
  line L73 (2.55, 12.5) -> (3.05, 12.5085) construction
  line L74 (3.05, 12.5085) -> (3.05, 7.5) construction
  line L75 (2.55, 12.5) -> (16.95, 12.5) construction
  line L76 (16.95, 12.5) -> (17.45, 12.5) construction
  line L77 (17.45, 12.5) -> (17.45, 7.5) construction
  line L78 (17.45, 7.5) -> (16.95, 7.5) construction
  line L79 (16.95, 7.5) -> (16.95, 12.5) construction
  line L80 (17.45, 7.5) -> (16.95, 7.5)
  line L81 (16.95, 7.5) -> (16.95, 12.5)
  line L82 (16.95, 12.5) -> (17.45, 12.5)
  line L83 (17.45, 12.5) -> (17.45, 7.5)
  line L84 (3.05, 7.5) -> (2.55, 7.5)
  line L85 (2.55, 7.5) -> (2.55, 12.5)
  line L86 (2.55, 12.5) -> (3.05, 12.5)
  line L87 (3.05, 12.5) -> (3.05, 7.5)
  dimension "d1_3" = 20
  dimension "d2_3" = 20
  dimension "d3_3" = 8.9
  dimension "d4_3" = 8.9
  dimension "d5_3" = 8.9
  dimension "d6_3" = 17.8
  dimension "d7_3" = 17.8
  dimension "d8_3" = 6.95
  dimension "d9_3" = 6.95
  dimension "d10_3" = 13.9
  dimension "d11_3" = 13.9
  dimension "d12_3" = 13.9
  dimension "d13_3" = 3
  dimension "d14_3" = 3
  dimension "d15_3" = 3
  dimension "d16_3" = 3
  dimension "d21_6" = 3
  dimension "d58_6" = 2.5
  dimension "d59_6" = 0.5
  dimension "d60_6" = 5
  dimension "d61_6" = 0.5
  dimension "d62_6" = 5
  constraint coincident L0.start L3.end
  constraint vertical L0
  constraint perpendicular L0 L1
  constraint perpendicular L1 L2
  constraint perpendicular L0 L3
  constraint midpoint L3 L6.start
  constraint parallel L3 L6
  constraint midpoint L4 L7.start
  constraint parallel L6 L7
  constraint perpendicular L7 L8
  constraint perpendicular L8 L9
  constraint perpendicular L9 L10
  constraint coincident L5 L11.end
  constraint perpendicular L10 L11
  constraint perpendicular L12 L13
  constraint perpendicular L13 L14
  constraint perpendicular L14 L15
  constraint perpendicular L7 L16
  constraint perpendicular L16 L17
  constraint coincident L0 L19.end
  constraint perpendicular L0 L19
  constraint coincident L3 L20.end
  constraint perpendicular L3 L20
  constraint coincident L2 L21.end
  constraint perpendicular L2 L21
  constraint coincident L2 L22.end
  constraint perpendicular L2 L22
  constraint coincident L1 L23.end
  constraint perpendicular L1 L23
  constraint coincident L1 L24.end
  constraint perpendicular L1 L24
  constraint coincident L0 L25.end
  constraint perpendicular L0 L25
  constraint coincident L24 L26.start
  constraint coincident L9 L26.start
  constraint coincident L9 L26.end
  constraint coincident L1 L27.end
  constraint perpendicular L1 L27
  constraint coincident L9 L28.start
  constraint coincident L23 L28.start
  constraint perpendicular L23 L28
  constraint coincident L1 L29.end
  constraint perpendicular L1 L29
  constraint coincident L6 L30.end
  constraint coincident L30 L31.start
  constraint coincident L11 L31.start
  constraint perpendicular L30 L31
  constraint coincident L6 L32.end
  constraint coincident L11 L33.start
  constraint coincident L20 L33.start
  constraint perpendicular L20 L33
  constraint coincident L3 L34.end
  constraint perpendicular L3 L34
  constraint horizontal L35
  constraint vertical L36
  constraint horizontal L37
  constraint vertical L38
  constraint horizontal L39
  constraint vertical L40
  constraint horizontal L41
  constraint vertical L42
  constraint horizontal L43
  constraint vertical L44
  constraint horizontal L45
  constraint vertical L46
  constraint horizontal L47
  constraint vertical L48
  constraint horizontal L49
  constraint vertical L50
  constraint horizontal L51
  constraint vertical L52
  constraint horizontal L53
  constraint vertical L54
  constraint horizontal L55
  constraint vertical L56
  constraint horizontal L57
  constraint vertical L58
  constraint horizontal L59
  constraint vertical L60
  constraint horizontal L61
  constraint vertical L62
  constraint midpoint L10 L63.start
  constraint coincident L10 L63.end
  constraint parallel L10 L63
  constraint coincident L10 L64.end
  constraint perpendicular L0 L65
  constraint horizontal L66
  constraint vertical L67
  constraint horizontal L68
  constraint vertical L69
  constraint perpendicular L13 L70
  constraint perpendicular L70 L71
  constraint perpendicular L71 L72
  constraint coincident L14 L73.end
  constraint perpendicular L71 L74
  constraint coincident L16 L75.end
  constraint perpendicular L16 L75
  constraint perpendicular L16 L76
  constraint perpendicular L76 L77
  constraint coincident L16 L78.end
  constraint perpendicular L16 L78
  constraint horizontal L80
  constraint vertical L81
  constraint horizontal L82
  constraint vertical L83
  constraint horizontal L84
  constraint vertical L85
  constraint horizontal L86
  constraint vertical L87
  measures "d1_3" distance of L0.start L0.end
  measures "d2_3" distance of L0.end L1.end
  measures "d3_3" distance of L6.start L6.end
  measures "d4_3" distance of L7.start L7.end
  measures "d5_3" distance of L7.end L8.end
  measures "d6_3" distance of L8.end L9.end
  measures "d7_3" distance of L9.end L10.end
  measures "d8_3" distance of L7.start L13.end
  measures "d9_3" distance of L13.end L14.end
  measures "d10_3" distance of L14.end L15.end
  measures "d11_3" distance of L15.end L16.end
  measures "d12_3" distance of L16.end L17.end
  measures "d13_3" distance of L26.start L26.end
  measures "d14_3" distance of L28.start L28.end
  measures "d15_3" distance of L31.start L31.end
  measures "d16_3" distance of L33.start L33.end
  measures "d21_6" distance of L64.end L65.end
  measures "d58_6" distance of L13.end L70.end
  measures "d59_6" distance of L70.end L71.end
  measures "d60_6" distance of L71.end L72.end
  measures "d61_6" distance of L75.end L76.end
  measures "d62_6" distance of L76.end L77.end
extrude "Extrude3'''''" add sketch "Sketch1 (13)" along normal blind 7.5 separate body contours L42 L63 L64 L65 L66 L67 L68 | L42 L65 L66 L68 L69 makes body 19 in component "main-switchbody (3)"
extrude "Extrude2'''''" add sketch "Sketch1 (13)" along normal blind 4 separate body contours L39 L40 L41 L42 L47 L48 L50 L51 L52 L54 L56 L57 L58 L60 L61 L62 L63 L64 L65 L66 L67 L68 | L42 L63 L64 L65 L66 L67 L68 | L46 L80 L81 L82 L83 | L44 L84 L85 L86 L87 makes body 20 in component "main-switchbody (3)"
extrude "Extrude1''''''''" add sketch "Sketch1 (13)" along normal blind 6 separate body contours L39 L59 L60 L61 L62 | L39 L55 L56 L57 L58 | L41 L47 L48 L49 L50 | L41 L51 L52 L53 L54 makes body 21 at (4.05, 1.1, 2) makes body 22 at (5.05, 20, 4) makes body 23 at (14.95, 1.1, 2) makes body 24 at (14.95, 20, 2) in component "main-switchbody (3)"
extrude "Extrude4''" cut sketch "Sketch1 (13)" along normal blind 2 contours L42 L65 L66 L68 L69 bodies 19 in component "main-switchbody (3)"
sketch "Sketch2 (10)" plane through (1.1, 0, 0) normal (1, 0, 0) x (0, 1, 0) in component "main-switchbody (3)"
  line L0 (8, 0) -> (12, 0)
  line L1 (12, 0) -> (12, 7.5)
  line L2 (12, 7.5) -> (8, 7.5)
  line L3 (8, 7.5) -> (8, 0)
  line L4 (8, 7.5) -> (8, 4) construction
  line L5 (8, 4) -> (12, 4) construction
  line L6 (12, 4) -> (12, 7.5) construction
  line L7 (12, 7.5) -> (8, 7.5) construction
  line L8 (8, 7.5) -> (8, 5.75) construction
  line L9 (8, 5.75) -> (12, 5.75) construction
  line L10 (8, 7.5) -> (12, 7.5)
  line L11 (12, 7.5) -> (12, 5.75)
  line L12 (12, 5.75) -> (8, 5.75)
  line L13 (8, 5.75) -> (8, 7.5)
  dimension "d26_6" = 1.75
  constraint coincident L2.end L3.start
  constraint coincident L3 L4.end
  constraint perpendicular L2 L4
  constraint coincident L1 L5.end
  constraint perpendicular L1 L5
  constraint coincident L1.end L2.start
  constraint perpendicular L2 L6
  constraint perpendicular L5 L8
  constraint midpoint L6 L9.end
  constraint horizontal L10
  constraint vertical L11
  constraint horizontal L12
  constraint vertical L13
  measures "d26_6" distance of L2.end L8.end
extrude "Extrude5''" add sketch "Sketch2 (10)" along normal blind 1 contours L1 L2 L3 L10 L11 L12 L13 bodies 19 in component "main-switchbody (3)"
extrude "Extrude6''" cut 1 faces at (-1.9, 10.6667, 3.8333) along direction (1, 0, 0) blind 1 on bodies 19 bodies 19 in component "main-switchbody (3)"
sketch "Sketch3 (3)" plane through (0, 18.9, 0) normal (0, -1, 0) x (1, 0, 0) in component "main-switchbody (3)"
  line L0 (3.05, 0) -> (6.05, 0)
  line L1 (6.05, 0) -> (6.05, 6)
  line L2 (6.05, 6) -> (3.05, 6)
  line L3 (3.05, 6) -> (3.05, 0)
  line L4 (3.05, 6) -> (3.05, 4) construction
  line L5 (6.05, 4) -> (6.05, 6) construction
  line L6 (3.05, 6) -> (3.05, 4.5) construction
  line L7 (6.05, 6) -> (6.05, 4.5) construction
  arc A0 (6.05, 4.5) -> (3.05, 4.5) centre (4.55, 4.5) ccw construction
  arc A1 (6.05, 4.5) -> (3.05, 4.5) centre (4.55, 4.5) ccw
  dimension "d31_6" = 1.5
  dimension "d32_6" = 1.5
  constraint coincident L2.end L3.start
  constraint coincident L3 L4.end
  constraint perpendicular L2 L4
  constraint coincident L1 L5.start
  constraint coincident L1.end L2.start
  constraint perpendicular L2 L5
  constraint perpendicular L2 L6
  constraint perpendicular L2 L7
  constraint tangent L2 A0
  constraint tangent L2 A1
  measures "d31_6" distance of L2.end L6.end
  measures "d32_6" distance of L1.end L7.end
extrude "Extrude7''" cut sketch "Sketch3 (3)" against normal blind 1.1 contours L2 L3 A1 | L1 L2 A1 bodies 22 in component "main-switchbody (3)"
sketch "Sketch4 (3)" plane through (0, 0, 0) normal (0, -1, 0) x (1, 0, 0) in component "main-switchbody (3)"
  line L0 (3.05, 0) -> (6.05, 0)
  line L1 (6.05, 0) -> (6.05, 6)
  line L2 (6.05, 6) -> (3.05, 6)
  line L3 (3.05, 6) -> (3.05, 0)
  line L4 (3.05, 6) -> (3.05, 4.5) construction
  line L5 (6.05, 6) -> (6.05, 4.5) construction
  arc A0 (6.05, 4.5) -> (3.05, 4.5) centre (4.55, 4.5) ccw
  constraint coincident L2.end L3.start
  constraint coincident L3 L4.end
  constraint perpendicular L2 L4
  constraint coincident L1.end L2.start
  constraint coincident L1 L5.end
  constraint perpendicular L2 L5
  constraint tangent L2 A0
extrude "Extrude8''" cut sketch "Sketch4 (3)" against normal blind 1.1 contours L2 L3 A0 | L1 L2 A0 bodies 21 in component "main-switchbody (3)"
sketch "Sketch5 (3)" plane through (0, 0, 0) normal (0, -1, 0) x (1, 0, 0) in component "main-switchbody (3)"
  line L0 (13.95, 0) -> (16.95, 0)
  line L1 (16.95, 0) -> (16.95, 6)
  line L2 (16.95, 6) -> (13.95, 6)
  line L3 (13.95, 6) -> (13.95, 0)
  line L4 (13.95, 6) -> (13.95, 4.5) construction
  line L5 (16.95, 6) -> (16.95, 4.5) construction
  arc A0 (16.95, 4.5) -> (13.95, 4.5) centre (15.45, 4.5) ccw
  constraint coincident L2.end L3.start
  constraint coincident L3 L4.end
  constraint perpendicular L2 L4
  constraint coincident L1.end L2.start
  constraint coincident L1 L5.end
  constraint perpendicular L2 L5
  constraint tangent L2 A0
extrude "Extrude9''" cut sketch "Sketch5 (3)" against normal blind 1.1 contours L2 L3 A0 | L1 L2 A0 bodies 23 in component "main-switchbody (3)"